Odrive Rack_v2 (Autodesk Fusion 360 design; units mm, degrees)
Autodesk Fusion 360 part; units mm, degrees
sketch "Sketch1" plane through (0, 0, 0) normal (0, 0, 1) x (1, 0, 0)
  line L0 (0, 0) -> (37.5, 0)
  line L1 (37.5, 0) -> (37.5, 30)
  line L2 (0, 0) -> (37.5, 0) construction
  line L3 (37.5, 30) -> (42.5, 30)
  line L4 (42.5, 30) -> (42.5, -30)
  line L5 (42.5, -30) -> (122.5, -30)
  line L6 (122.5, -30) -> (122.5, -160)
  line L7 (122.5, -160) -> (0, -160)
  line L8 (0, 0) -> (0, -160)
  dimension "d1" = 37.5
  dimension "d2" = 30
  dimension "d3" = 5
  dimension "d4" = 60
  dimension "d5" = 80
  dimension "d6" = 130
  dimension "d7" = 122.5
  dimension "d8" = 190
  constraint horizontal L0
  constraint vertical L1
  constraint coincident L0.start L2.start
  constraint perpendicular L1 L3
  constraint perpendicular L4 L5
  constraint perpendicular L5 L6
  constraint perpendicular L6 L7
  constraint perpendicular L7 L8
  measures "d1" distance of L0.start L0.end
  measures "d2" distance of L0.end L1.end
  measures "d3" distance of L1.end L3.end
  measures "d4" distance of L3.end L4.end
  measures "d5" distance of L4.end L5.end
  measures "d6" distance of L5.end L6.end
  measures "d7" distance of L6.end L7.end
  measures "d8" distance of L3 L7
extrude "Extrude1" add sketch "Sketch1" along normal blind 5
mirror "Mirror1" about plane through (0, 0, 0) normal (1, 0, 0) of bodies 1 merged
sketch "Sketch3" plane through (0, 0, 5) normal (0, 0, 1) x (-1, 0, 0)
  line L0 (-37.5, 0) -> (37.5, 0)
  line L1 (122.5, 160) -> (-122.5, 160)
  line L2 (-122.5, 160) -> (-122.5, 30)
  line L3 (-122.5, 30) -> (-42.5, 30)
  line L4 (-42.5, 30) -> (-42.5, -30)
  line L5 (-42.5, -30) -> (-37.5, -30)
  line L6 (-37.5, -30) -> (-37.5, 0)
  line L7 (-42.5, 30) -> (-52.5, 30) construction
  line L8 (-52.5, 30) -> (-52.5, 35) construction
  line L9 (-52.5, 35) -> (-42.5, 35) construction
  line L10 (-42.5, 35) -> (-42.5, 30) construction
  line L11 (-42.5, 30) -> (-77.5, 30) construction
  line L12 (-77.5, 30) -> (-77.5, 45) construction
  line L13 (-77.5, 45) -> (-42.5, 45) construction
  line L14 (-42.5, 45) -> (-42.5, 30) construction
  line L15 (-42.5, 30) -> (-102.5, 30) construction
  line L16 (-102.5, 30) -> (-102.5, 55) construction
  line L17 (-102.5, 55) -> (-42.5, 55) construction
  line L18 (-42.5, 55) -> (-42.5, 30) construction
  line L19 (-52.5, 35) -> (-54.5, 35)
  line L20 (-54.5, 35) -> (-54.5, 40)
  line L21 (-54.5, 40) -> (-52.5, 40)
  line L22 (-52.5, 40) -> (-52.5, 35)
  line L23 (-77.5, 45) -> (-79.5, 45)
  line L24 (-79.5, 45) -> (-79.5, 50)
  line L25 (-79.5, 50) -> (-77.5, 50)
  line L26 (-77.5, 50) -> (-77.5, 45)
  line L27 (-102.5, 55) -> (-104.5, 55)
  line L28 (-104.5, 55) -> (-104.5, 60)
  line L29 (-104.5, 60) -> (-102.5, 60)
  line L30 (-102.5, 60) -> (-102.5, 55)
  line L31 (-52.5, 40) -> (-54.5, 40) construction
  line L32 (-54.5, 40) -> (-54.5, 104.8)
  line L33 (-54.5, 104.8) -> (-52.5, 104.8) construction
  line L34 (-52.5, 104.8) -> (-52.5, 40)
  line L35 (-104.5, 60) -> (-102.5, 60) construction
  line L36 (-102.5, 60) -> (-102.5, 124.8)
  line L37 (-102.5, 124.8) -> (-104.5, 124.8) construction
  line L38 (-104.5, 124.8) -> (-104.5, 60)
  line L39 (-77.5, 50) -> (-79.5, 50) construction
  line L40 (-79.5, 50) -> (-79.5, 114.8)
  line L41 (-79.5, 114.8) -> (-77.5, 114.8) construction
  line L42 (-77.5, 114.8) -> (-77.5, 50)
  line L43 (-52.5, 104.8) -> (-54.5, 104.8)
  line L44 (-54.5, 104.8) -> (-54.5, 109.8)
  line L45 (-54.5, 109.8) -> (-52.5, 109.8)
  line L46 (-52.5, 109.8) -> (-52.5, 104.8)
  line L47 (-77.5, 114.8) -> (-79.5, 114.8)
  line L48 (-79.5, 114.8) -> (-79.5, 119.8)
  line L49 (-79.5, 119.8) -> (-77.5, 119.8)
  line L50 (-77.5, 119.8) -> (-77.5, 114.8)
  line L51 (-102.5, 124.8) -> (-104.5, 124.8)
  line L52 (-104.5, 124.8) -> (-104.5, 129.8)
  line L53 (-104.5, 129.8) -> (-102.5, 129.8)
  line L54 (-102.5, 129.8) -> (-102.5, 124.8)
  line L55 (37.5, 0) -> (37.5, -30)
  line L56 (37.5, -30) -> (42.5, -30)
  line L57 (42.5, -30) -> (42.5, 30)
  line L58 (42.5, 30) -> (122.5, 30)
  line L59 (122.5, 30) -> (122.5, 160)
  dimension "d39" = 10
  dimension "d40" = 5
  dimension "d41" = 35
  dimension "d42" = 15
  dimension "d46" = 60
  dimension "d47" = 25
  dimension "d48" = 2
  dimension "d49" = 5
  dimension "d50" = 2
  dimension "d51" = 5
  dimension "d52" = 2
  dimension "d53" = 5
  dimension "d54" = 2
  dimension "d55" = 64.8
  dimension "d58" = 2
  dimension "d59" = 64.8
  dimension "d60" = 2
  dimension "d61" = 64.8
  dimension "d62" = 2
  dimension "d63" = 5
  dimension "d64" = 2
  dimension "d65" = 5
  dimension "d66" = 2
  dimension "d67" = 5
  constraint horizontal L7
  constraint vertical L8
  constraint horizontal L9
  constraint vertical L10
  constraint coincident L3.end L4.start
  constraint horizontal L11
  constraint vertical L12
  constraint horizontal L13
  constraint vertical L14
  constraint horizontal L15
  constraint vertical L16
  constraint horizontal L17
  constraint vertical L18
  constraint horizontal L19
  constraint vertical L20
  constraint horizontal L21
  constraint vertical L22
  constraint horizontal L23
  constraint vertical L24
  constraint horizontal L25
  constraint vertical L26
  constraint horizontal L27
  constraint vertical L28
  constraint horizontal L29
  constraint vertical L30
  constraint horizontal L31
  constraint vertical L32
  constraint horizontal L33
  constraint vertical L34
  constraint horizontal L35
  constraint vertical L36
  constraint horizontal L37
  constraint vertical L38
  constraint horizontal L39
  constraint vertical L40
  constraint horizontal L41
  constraint vertical L42
  constraint horizontal L43
  constraint vertical L44
  constraint horizontal L45
  constraint vertical L46
  constraint horizontal L47
  constraint vertical L48
  constraint horizontal L49
  constraint vertical L50
  constraint horizontal L51
  constraint vertical L52
  constraint horizontal L53
  constraint vertical L54
  measures "d39" distance of L3.end L7.end
  measures "d40" distance of L3.end L9.end
  measures "d41" distance of L3.end L11.end
  measures "d42" distance of L3.end L13.end
  measures "d46" distance of L3.end L15.end
  measures "d47" distance of L3.end L17.end
  measures "d48" distance of L8.end L19.end
  measures "d49" distance of L8.end L21.end
  measures "d50" distance of L12.end L23.end
  measures "d51" distance of L12.end L25.end
  measures "d52" distance of L16.end L27.end
  measures "d53" distance of L16.end L29.end
  measures "d54" distance of L21.end L20.end
  measures "d55" distance of L21.end L33.end
  measures "d58" distance of L28.end L29.end
  measures "d59" distance of L28.end L37.end
  measures "d60" distance of L25.end L24.end
  measures "d61" distance of L25.end L41.end
  measures "d62" distance of L33.end L32.end
  measures "d63" distance of L33.end L45.end
  measures "d64" distance of L41.end L40.end
  measures "d65" distance of L41.end L49.end
  measures "d66" distance of L36.end L37.end
  measures "d67" distance of L36.end L53.end
extrude "Extrude2" add sketch "Sketch3" along normal blind 55 contours L19 L20 L21 L22 | L43 L44 L45 L46 | L23 L24 L25 L26 | L47 L48 L49 L50 | L27 L28 L29 L30 | L51 L52 L53 L54
fillet "Fillet1" radius 4 12 edges at (52.5, -37.5, 5) (52.5, -107.3, 5) (77.5, -117.3, 5) (102.5, -127.3, 5) (102.5, -57.5, 5) (77.5, -47.5, 5) (54.5, -107.3, 5) (79.5, -117.3, 5) (104.5, -127.3, 5) (104.5, -57.5, 5) (79.5, -47.5, 5) (54.5, -37.5, 5)
fillet "Fillet2" radius 4 6 edges at (78.5, -119.8, 5) (103.5, -129.8, 5) (53.5, -109.8, 5) (103.5, -55, 5) (78.5, -45, 5) (53.5, -35, 5)
sketch "Sketch4" plane through (52.5, 0, 0) normal (-1, 0, 0) x (0, -1, 0)
  line L0 (35, 9) -> (40, 9)
  line L1 (40, 9) -> (40, 60)
  line L2 (40, 60) -> (35, 60)
  line L3 (35, 60) -> (35, 9)
  line L4 (35, 60) -> (42.5, 60)
  line L5 (42.5, 60) -> (42.5, 35)
  line L6 (42.5, 35) -> (35, 35)
  line L7 (35, 35) -> (35, 60)
  line L8 (109.8, 60) -> (102.3, 60)
  line L9 (102.3, 60) -> (102.3, 35)
  line L10 (102.3, 35) -> (109.8, 35)
  line L11 (109.8, 35) -> (109.8, 60)
  line L12 (45, 60, -25) -> (52.5, 60, -25)
  line L13 (52.5, 60, -25) -> (52.5, 35, -25)
  line L14 (52.5, 35, -25) -> (45, 35, -25)
  line L15 (45, 35, -25) -> (45, 60, -25)
  line L16 (55, 60, -50) -> (62.5, 60, -50)
  line L17 (62.5, 60, -50) -> (62.5, 35, -50)
  line L18 (62.5, 35, -50) -> (55, 35, -50)
  line L19 (55, 35, -50) -> (55, 60, -50)
  line L20 (119.8, 60, -25) -> (112.3, 60, -25)
  line L21 (112.3, 60, -25) -> (112.3, 35, -25)
  line L22 (112.3, 35, -25) -> (119.8, 35, -25)
  line L23 (119.8, 35, -25) -> (119.8, 60, -25)
  line L24 (129.8, 60, -50) -> (122.3, 60, -50)
  line L25 (122.3, 60, -50) -> (122.3, 35, -50)
  line L26 (122.3, 35, -50) -> (129.8, 35, -50)
  line L27 (129.8, 35, -50) -> (129.8, 60, -50)
  point P0 (109.8, 60)
  point P1 (45, 60)
  point P2 (55, 60)
  point P3 (119.8, 60)
  point P4 (129.8, 60)
  dimension "d74" = 7.5
  dimension "d75" = 25
  dimension "d76" = 7.5
  dimension "d77" = 25
  dimension "d78" = 7.5
  dimension "d79" = 25
  dimension "d80" = 7.5
  dimension "d81" = 25
  dimension "d82" = 7.5
  dimension "d83" = 25
  dimension "d84" = 7.5
  dimension "d85" = 25
  constraint horizontal L4
  constraint vertical L5
  constraint horizontal L6
  constraint vertical L7
  constraint coincident L2.end L3.start
  constraint horizontal L8
  constraint vertical L9
  constraint horizontal L10
  constraint vertical L11
  constraint coincident P0 L8.start
  measures "d74" distance of L2.end L4.end
  measures "d75" distance of L2.end L6.end
  measures "d76" distance of P0 L8.end
  measures "d77" distance of P0 L10.end
extrude "Extrude3" add sketch "Sketch4" along normal blind 3 contours L1 L2 L3 L4 L6 L7 | L1 L4 L5 L6 | L8 L9 L10 L11
extrude "Extrude4" add sketch "Sketch4" along normal blind 3 contours L12 L13 L14 L15 | L20 L21 L22 L23 in plane through (77.5, 0, 0) normal (-1, 0, 0)
extrude "Extrude5" add sketch "Sketch4" along normal blind 3 contours L16 L17 L18 L19 | L24 L25 L26 L27 in plane through (102.5, 0, 0) normal (-1, 0, 0)
extrude "Extrude6" add sketch "Sketch4" against normal blind 5 contours L1 L2 L3 L4 L6 L7 | L1 L4 L5 L6 | L8 L9 L10 L11
extrude "Extrude7" add sketch "Sketch4" against normal blind 5 contours L12 L13 L14 L15 | L20 L21 L22 L23 in plane through (77.5, 0, 0) normal (-1, 0, 0)
extrude "Extrude8" add sketch "Sketch4" against normal blind 5 contours L16 L17 L18 L19 | L24 L25 L26 L27 in plane through (102.5, 0, 0) normal (-1, 0, 0)
pattern_linear "R-Pattern1" count 2 spacing 160 along (-1, 0, 0) of "Extrude2", "Fillet1", "Fillet2", "Extrude3", "Extrude4", "Extrude5", "Extrude6", "Extrude7", "Extrude8"
extrude "Extrude9" cut sketch "Sketch3" along normal blind 66 contours L21 L32 L34 L43 | L25 L40 L42 L47 | L29 L36 L38 L51
sketch "Sketch5" plane through (0, 0, 5) normal (0, 0, 1) x (-1, 0, 0)
  line L0 (-48.5, 104.8) -> (-58.5, 104.8)
  line L1 (-58.5, 104.8) -> (-58.5, 113.8)
  line L2 (-58.5, 113.8) -> (-48.5, 113.8)
  line L3 (-48.5, 113.8) -> (-48.5, 104.8)
  line L4 (-73.5, 114.8) -> (-83.5, 114.8)
  line L5 (-83.5, 114.8) -> (-83.5, 123.8)
  line L6 (-83.5, 123.8) -> (-73.5, 123.8)
  line L7 (-73.5, 123.8) -> (-73.5, 114.8)
  line L8 (-108.5, 60) -> (-98.5, 60)
  line L9 (-98.5, 60) -> (-98.5, 51)
  line L10 (-98.5, 51) -> (-108.5, 51)
  line L11 (-108.5, 51) -> (-108.5, 60)
  line L12 (-58.5, 40) -> (-48.5, 40)
  line L13 (-48.5, 40) -> (-48.5, 31)
  line L14 (-48.5, 31) -> (-58.5, 31)
  line L15 (-58.5, 31) -> (-58.5, 40)
  line L16 (-83.5, 50) -> (-73.5, 50)
  line L17 (-73.5, 50) -> (-73.5, 41)
  line L18 (-73.5, 41) -> (-83.5, 41)
  line L19 (-83.5, 41) -> (-83.5, 50)
  line L20 (-98.5, 124.8) -> (-108.5, 124.8)
  line L21 (-108.5, 124.8) -> (-108.5, 133.8)
  line L22 (-108.5, 133.8) -> (-98.5, 133.8)
  line L23 (-98.5, 133.8) -> (-98.5, 124.8)
  line L24 (101.5, 31) -> (101.5, 40)
  line L25 (101.5, 40) -> (111.5, 40)
  line L26 (111.5, 40) -> (111.5, 31)
  line L27 (111.5, 31) -> (101.5, 31)
  line L28 (76.5, 41) -> (76.5, 50)
  line L29 (76.5, 50) -> (86.5, 50)
  line L30 (86.5, 50) -> (86.5, 41)
  line L31 (86.5, 41) -> (76.5, 41)
  line L32 (51.5, 51) -> (51.5, 60)
  line L33 (51.5, 60) -> (61.5, 60)
  line L34 (61.5, 60) -> (61.5, 51)
  line L35 (61.5, 51) -> (51.5, 51)
  line L36 (111.5, 113.8) -> (111.5, 104.8)
  line L37 (111.5, 104.8) -> (101.5, 104.8)
  line L38 (101.5, 104.8) -> (101.5, 113.8)
  line L39 (101.5, 113.8) -> (111.5, 113.8)
  line L40 (61.5, 133.8) -> (61.5, 124.8)
  line L41 (61.5, 124.8) -> (51.5, 124.8)
  line L42 (51.5, 124.8) -> (51.5, 133.8)
  line L43 (51.5, 133.8) -> (61.5, 133.8)
  line L44 (86.5, 123.8) -> (86.5, 114.8)
  line L45 (86.5, 114.8) -> (76.5, 114.8)
  line L46 (76.5, 114.8) -> (76.5, 123.8)
  line L47 (76.5, 123.8) -> (86.5, 123.8)
  line L48 (-37.5, 0) -> (37.5, 0)
  line L49 (37.5, 0) -> (37.5, -30)
  line L50 (37.5, -30) -> (42.5, -30)
  line L51 (42.5, -30) -> (42.5, 30)
  line L52 (42.5, 30) -> (122.5, 30)
  line L53 (122.5, 30) -> (122.5, 160)
  line L54 (122.5, 160) -> (-122.5, 160)
  line L55 (-122.5, 160) -> (-122.5, 30)
  line L56 (-122.5, 30) -> (-42.5, 30)
  line L57 (-42.5, 30) -> (-42.5, -30)
  line L58 (-42.5, -30) -> (-37.5, -30)
  line L59 (-37.5, -30) -> (-37.5, 0)
  line L60 (106.5, 40) -> (107.5, 40) construction
  line L61 (81.5, 50) -> (82.5, 50) construction
  line L62 (56.5, 60) -> (57.5, 60) construction
  line L63 (107.5, 40) -> (105.5, 40)
  line L64 (105.5, 40) -> (105.5, 104.8)
  line L65 (105.5, 104.8) -> (107.5, 104.8)
  line L66 (107.5, 104.8) -> (107.5, 40)
  line L67 (82.5, 50) -> (80.5, 50)
  line L68 (80.5, 50) -> (80.5, 114.8)
  line L69 (80.5, 114.8) -> (82.5, 114.8)
  line L70 (82.5, 114.8) -> (82.5, 50)
  line L71 (57.5, 60) -> (55.5, 60)
  line L72 (55.5, 60) -> (55.5, 124.8)
  line L73 (55.5, 124.8) -> (57.5, 124.8)
  line L74 (57.5, 124.8) -> (57.5, 60)
  dimension "d106" = 1
  dimension "d107" = 1
  dimension "d108" = 1
  dimension "d109" = 2
  dimension "d110" = 64.8
  dimension "d111" = 2
  dimension "d112" = 64.8
  dimension "d113" = 2
  dimension "d114" = 64.8
  constraint midpoint L25 L60.start
  constraint parallel L25 L60
  constraint midpoint L29 L61.start
  constraint parallel L29 L61
  constraint midpoint L33 L62.start
  constraint parallel L33 L62
  constraint horizontal L63
  constraint vertical L64
  constraint horizontal L65
  constraint vertical L66
  constraint vertical L68
  constraint perpendicular L67 L68
  constraint horizontal L69
  constraint vertical L70
  constraint horizontal L71
  constraint vertical L72
  constraint horizontal L73
  constraint vertical L74
  measures "d106" distance of L60.start L60.end
  measures "d107" distance of L61.start L61.end
  measures "d108" distance of L62.start L62.end
  measures "d109" distance of L60.end L63.end
  measures "d110" distance of L60.end L65.end
  measures "d111" distance of L61.end L67.end
  measures "d112" distance of L61.end L69.end
  measures "d113" distance of L62.end L71.end
  measures "d114" distance of L62.end L73.end
extrude "Extrude10" cut sketch "Sketch5" along normal blind 76 contours L25 L37 L63 L64 L65 L66 | L29 L45 L67 L68 L69 L70 | L33 L41 L71 L72 L73 L74
equation "d1 = ( 75 / 2 ) * 1 mm"
equation "d7 = d1 + d3 + d5"
equation "d41 = OdriveWidth + d39"
equation "d42 = OdriveOffset + d40"
equation "OdriveWidth = 25 mm"
equation "OdriveLength = 64.8 mm"
equation "OdriveOffset = 10 mm"
equation "d46 = OdriveWidth + d41"
equation "d47 = OdriveOffset + d42"
equation "d55 = OdriveLength"
equation "d59 = OdriveLength"
equation "d61 = OdriveLength"
equation "d76 = d74"
equation "d77 = d75"
equation "d78 = d74"
equation "d79 = d75"
equation "d80 = d74"
equation "d81 = d75"
equation "d82 = d74"
equation "d83 = d75"
equation "d84 = d74"
equation "d85 = d75"
equation "d110 = OdriveLength"
equation "d112 = OdriveLength"
equation "d114 = OdriveLength"
